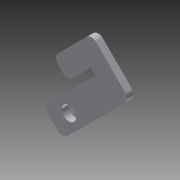
# Autodesk Inventor part: V5 Conveyor Plate Bracket P3
Saved by Autodesk Inventor 2014 SP1 (Build 180222100, 222)
## iProperties
Created: 2012-02-17
Part Number: V5 Conveyor Plate Bracket P3
Material: Aluminum-6061
Document SubType Name: Modeling
Designer: Moses
Mass: 6.79011 g
Surface Area: 21.615 cm^2
Volume: 2.50558 cm^3
Density: 2.71 g/cm^3
Appearance: Aluminum - Flat
Author: Moses
Autodesk Inventor part; units mm, degrees
ref_plane "YZ Plane" through (0, 0, 0) normal (1, 0, 0) x (0, 1, 0)
ref_plane "XZ Plane" through (0, 0, 0) normal (0, 1, 0) x (-1, 0, 0)
ref_plane "XY Plane" through (0, 0, 0) normal (0, 0, 1) x (1, 0, 0)
sketch "Sketch1" plane through (0, 0, 0) normal (0, 0, 1) x (1, 0, 0)
  line L0 (-53.3927, 155.3954) -> (-51.1476, 153.1504) construction
  line L1 (-53.3927, 155.3954) -> (-73.3092, 135.4789) construction
  line L2 (-73.3092, 135.4789) -> (-71.0641, 133.2339) construction
  line L3 (-71.0641, 133.2339) -> (-51.1476, 153.1504) construction
  line L4 (-46.6575, 157.6405) -> (-51.1476, 153.1504) construction
  line L5 (-46.6575, 157.6405) -> (-48.9026, 159.8856) construction
  line L6 (-53.3927, 155.3954) -> (-48.9026, 159.8856) construction
  line L7 (-59.8388, 148.9493) -> (-66.574, 155.6845)
  line L8 (-66.574, 155.6845) -> (-48.6135, 173.645)
  line L9 (-48.6135, 173.645) -> (-30.653, 155.6845)
  line L10 (-30.653, 155.6845) -> (-62.0839, 124.2536)
  line L11 (-62.0839, 124.2536) -> (-71.0641, 133.2339)
  line L12 (-59.8388, 148.9493) -> (-48.9026, 159.8856)
  line L13 (-48.9026, 159.8856) -> (-46.6575, 157.6405)
  line L14 (-46.6575, 157.6405) -> (-71.0641, 133.2339)
  circle A0 centre (-59.164, 136.1538) radius 3.3782 projected
  point P0 (0, 0)
  dimension "d7" = 44.45
  dimension "d8" = 25.4
  dimension "d9" = 25.4
  dimension "d10" = 12.7
  constraints: 16 end point, 6 perpendicular, 2 parallel, 1 collinear, 1 point on line
  measures "d7" distance of L9.end L10.end
  measures "d8" distance of L8.end L9.end
  measures "d9" distance of L7.end L8.end
  measures "d10" distance of L10.end L2.end
extrude "Extrusion1" add sketch "Sketch1" along normal blind 3.175
fillet "Fillet1" radius 3.175 6 edges at (-62.0839, 124.2536, 1.5875) (-59.8388, 148.9493, 1.5875) (-66.574, 155.6845, 1.5875) (-71.0641, 133.2339, 1.5875) (-48.6135, 173.645, 1.5875) (-30.653, 155.6845, 1.5875)
body "Solid1"
